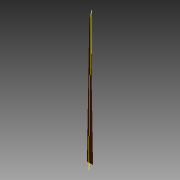
# Autodesk Inventor part: octoBotoStemRibSectA_V01
Saved by Autodesk Inventor 2013 (Build 170138000, 138)
## iProperties
Created: 2014-08-26
Part Number: octoBotoStemRibSectA_V01
Material: Wood (Walnut)
Document SubType Name: Modeling
Designer: Nano
Density: 0.55 g/cm^3
Mass: 117.319 g
Surface Area: 519.234 cm^2
Volume: 213.308 cm^3
Author: Nano
Autodesk Inventor part; units mm, degrees
ref_plane "YZ Plane" through (0, 0, 0) normal (1, 0, 0) x (0, 1, 0)
ref_plane "XZ Plane" through (0, 0, 0) normal (0, 1, 0) x (-1, 0, 0)
ref_plane "XY Plane" through (0, 0, 0) normal (0, 0, 1) x (1, 0, 0)
sketch "Sketch1" plane through (0, 0, 0) normal (0, 0, 1) x (1, 0, 0)
  line L0 (-1.5875, 9.6268) -> (1.5875, 9.6268)
  line L1 (1.5875, 9.6268) -> (12.7, -587.2732)
  line L2 (12.7, -587.2732) -> (-12.7, -587.2732)
  line L3 (-12.7, -587.2732) -> (-1.5875, 9.6268)
  line L4 (0, -13.6891) -> (0, 13.6891) construction
  line L5 (-3.175, -75.6446) -> (3.175, -75.6446) construction
  line L6 (0, 9.6268) -> (0, -588.1803) construction
  circle A0 centre (0, -580.9232) radius 1.651
  circle A1 centre (0, -574.5732) radius 1.651
  circle A2 centre (0, -568.2232) radius 1.651
  circle A3 centre (0, -561.8732) radius 1.651
  circle A4 centre (0, -555.5232) radius 1.651
  circle A5 centre (-6.35, -580.9232) radius 1.651
  circle A6 centre (-6.35, -574.5732) radius 1.651
  circle A7 centre (-6.35, -568.2232) radius 1.651
  circle A8 centre (-6.35, -561.8732) radius 1.651
  circle A9 centre (-6.35, -555.5232) radius 1.651
  circle A10 centre (6.35, -580.9232) radius 1.651
  circle A11 centre (6.35, -574.5732) radius 1.651
  circle A12 centre (6.35, -568.2232) radius 1.651
  circle A13 centre (6.35, -561.8732) radius 1.651
  circle A14 centre (6.35, -555.5232) radius 1.651
  line L7 (-3.1159, -72.4696) -> (3.1159, -72.4696) construction
  circle A15 centre (0, -71.7076) radius 0.762
  point P0 (0, 0)
  point P1 (0, 0)
  dimension "d0" = 3.175
  dimension "d9" = 596.9
  dimension "d10" = 25.4
  dimension "d11" = 6.35
  dimension "d12" = 1.5875
  dimension "d13" = 1.5875
  dimension "d14" = 3.302
  dimension "d15" = 6.35
  dimension "d18" = 6.35
  dimension "d21" = 6.35
  dimension "d26" = 6.35
  dimension "d34" = 3.175
  dimension "d35" = 1.524
  constraints: 16 centre point, 16 end point, 4 point on line, 3 parallel, 2 horizontal, 2 vertical, 1 coincident, 1 collinear, 1 equal length, 1 midpoint, 1 perpendicular, 1 tangent, 28 other
  measures "d0" distance of L0.end L0.start
  measures "d9" distance between parallel lines of L2 L0
  measures "d10" distance of L1.end L2.end
  measures "d11" distance of L5.start L5.end
  measures "d12" distance of L0.start L6.start
  measures "d13" distance of L0.end L6.start
  measures "d14" diameter of A0
  measures "d15" distance from line of L2 A0.centre
  measures "d18" distance of A0.centre A1.centre
  measures "d21" distance of A0.centre A5.centre
  measures "d26" distance of A0.centre A10.centre
  measures "d34" distance between parallel lines of L5 L7
  measures "d35" diameter of A15
extrude "Extrusion2" add sketch "Sketch1" along normal blind 3.175
fillet "Fillet1" radius 1.524 2 edges at (1.5875, 9.6268, 1.5875) (-1.5875, 9.6268, 1.5875)
sketch "Sketch2" plane through (0, 0, 3.175) normal (0, 0, 1) x (1, 0, 0)
  line L0 (-12.7, -587.2732) -> (12.7, -587.2732) projected
  ellipse E0 centre (-3.81, -523.7732) end of major axis (-3.81, -517.4232) minor radius 1.5875
  line L1 (0, -587.2732) -> (0, 9.6268) construction
  ellipse E1 centre (3.81, -523.7732) end of major axis (3.81, -517.4232) minor radius 1.5875
  point P0 (0, 0)
  dimension "d39" = 6.35
  dimension "d40" = 1.5875
  dimension "d41" = 63.5
  dimension "d42" = 8.89
  constraints: 2 end point, 1 symmetric about line, 1 vertical, 4 other
  measures "d41" distance from line of L0 point (-3.81, -523.773)
  measures "d42" horizontal distance of L0.start point (-3.81, -523.773)
extrude "Extrusion3" cut sketch "Sketch2" against normal through all
ref_plane "Work Plane1" through (-3.81, -523.7732, 3.175) normal (-0.9998267, 0.0186138, 0) x (0, 0, 1)
equation "\"d13\" = d12"
body "Solid2"
